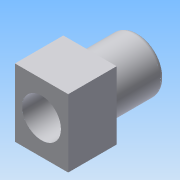
# Autodesk Inventor part: button
Saved by Autodesk Inventor 2015 (Build 190159000, 159)
## iProperties
Created: 2015-12-28
Part Number: button
Material: Générique
Document SubType Name: Modeling
Designer: Gregwar
Density: 1 g/cm^3
Appearance: Par défaut
Author: Gregwar
Autodesk Inventor part; units mm, degrees
ref_plane "YZ Plane" through (0, 0, 0) normal (1, 0, 0) x (0, 1, 0)
ref_plane "XZ Plane" through (0, 0, 0) normal (0, 1, 0) x (-1, 0, 0)
ref_plane "XY Plane" through (0, 0, 0) normal (0, 0, 1) x (1, 0, 0)
sketch "Esquisse1" plane through (0, 0, 0) normal (0, 1, 0) x (-1, 0, 0)
  circle A0 centre (0, 0) radius 2.75
  dimension "d0" = 5.5
  constraints: 1 centre point, 1 coincident
  measures "d0" diameter of A0
extrude "Extrusion1" add sketch "Esquisse1" along normal mid plane 10
sketch "Esquisse2" plane through (0, -5, 0) normal (0, -1, 0) x (1, 0, 0)
  circle A0 centre (0, 0) radius 2
  dimension "d3" = 4
  constraints: 1 centre point, 1 coincident
  measures "d3" diameter of A0
extrude "Extrusion2" cut sketch "Esquisse2" against normal blind 5
fillet "Congé1" radius 0.5 1 edges at (2.75, 5, 0)
sketch "Esquisse3" plane through (0, -5, 0) normal (0, -1, 0) x (1, 0, 0)
  line L0 (9.7978, 4.7343) -> (6.189, 4.7343)
  line L1 (6.189, 4.7343) -> (6.189, -4.7343)
  line L2 (6.189, -4.7343) -> (9.7978, -4.7343)
  line L3 (9.7978, -4.7343) -> (9.7978, 4.7343)
  circle A0 centre (0, 0) radius 2.75 projected
  line L4 (2.75, 0) -> (-2.75, 0) construction
  line L5 (9.7978, 0) -> (6.189, 0) construction
  line L6 (2.75, 3.5) -> (-2.75, 3.5)
  line L7 (-2.75, 3.5) -> (-2.75, -3.5)
  line L8 (-2.75, -3.5) -> (2.75, -3.5)
  line L9 (2.75, -3.5) -> (2.75, 3.5)
  line L10 (2.75, 0) -> (-2.75, 0) construction
  dimension "d7" = 5.5
  dimension "d8" = 5.5
  dimension "d9" = 7
  constraints: 22 end point, 4 midpoint, 4 parallel, 3 horizontal, 2 collinear, 2 perpendicular, 2 point on circle
  measures "d7" diameter of A0
  measures "d8" distance of L4.start L4.end
  measures "d9" distance between parallel lines of L6 L8
extrude "Extrusion3" add sketch "Esquisse3" against normal blind 5 contours L9 L8 L7 A0 | A0 L7 L6 L9
equation "\"d8\" = d7"
